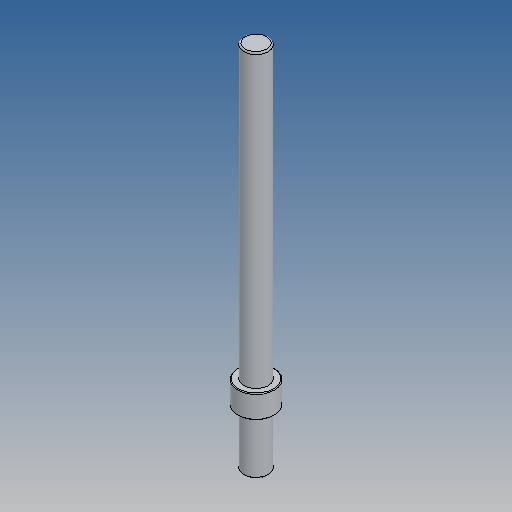
# Autodesk Inventor part: 63965-LtBluishGray
Saved by Autodesk Inventor 2025 (Build 290162010, 162A)
## iProperties
Created: 2014-06-21
Part Number: 63965-LtBluishGray
Material: ABS Plastic
Document SubType Name: Modeling
Designer: D. Kohfeld
Density: 1.06 g/cm^3
Appearance: LtBluishGray
Mass: 0.440924 g
Surface Area: 5.30755 cm^2
Volume: 0.415966 cm^3
Author: D. Kohfeld
Autodesk Inventor part; units mm, degrees
ref_plane "YZ Plane" through (0, 0, 0) normal (1, 0, 0) x (0, 1, 0)
ref_plane "XZ Plane" through (0, 0, 0) normal (0, 1, 0) x (-1, 0, 0)
ref_plane "XY Plane" through (0, 0, 0) normal (0, 0, 1) x (1, 0, 0)
sketch "Sketch1" plane through (0, 0, 0) normal (0, 0, 1) x (1, 0, 0)
  line L0 (0, -8.7) -> (1.6, -8.7)
  line L1 (1.6, -8.7) -> (1.6, -1.5)
  line L2 (1.6, -1.5) -> (2.4, -1.5)
  line L3 (2.4, -1.5) -> (2.4, 1.5)
  line L4 (2.4, 1.5) -> (1.6, 1.5)
  line L5 (1.6, 1.5) -> (1.6, 39.3)
  line L6 (1.6, 39.3) -> (0, 39.3)
  line L7 (0, 39.3) -> (0, -8.7)
  point P0 (0, 0)
  point P1 (2.4, 0)
  dimension "d1" = 48
  dimension "d2" = 3.2
  dimension "d3" = 3
  dimension "d4" = 4.8
  dimension "d5" = 7.2
  constraints: 16 end point, 5 parallel, 1 collinear, 1 horizontal, 1 horizontal alignment, 1 midpoint, 1 perpendicular, 1 point on line, 1 vertical alignment
  measures "d1" distance between parallel lines of L6 L0
  measures "d2" diameter of L5 L7
  measures "d3" distance of L2.end L3.end
  measures "d4" diameter of L3 L7
  measures "d5" distance between parallel lines of L0 L2
revolve "Revolution1" add sketch "Sketch1" angle 360 about axis through (0, 39.3, 0) along (0, -1, 0)
fillet "Fillet1" radius 0.1 2 edges at (-2.4, 1.5, 0) (-2.4, -1.5, 0)
fillet "Fillet1" radius 0.2 2 edges at (-1.6, 39.3, 0) (-1.6, -8.7, 0)
equation "\"d1\" = 6 * lu"
equation "\"d2\" = rd"
equation "\"d4\" = kd"
equation "\"d7\" = lf"
equation "\"lu\" = 8"
equation "\"rd\" = 3.2"
equation "\"kd\" = 4.8"
equation "\"lf\" = 0.1"
body "Solid1"
